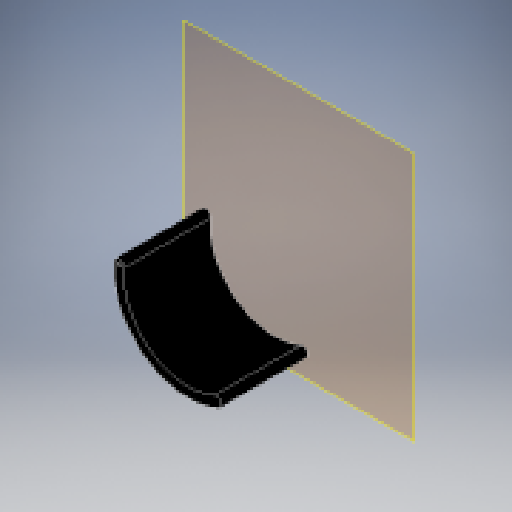
# Autodesk Inventor part: Mesh
Saved by Autodesk Inventor 2026.1 (Build 301233000, 233)
## iProperties
Created: 2025-09-20
Part Number: Mesh
Material: Generic
Document SubType Name: Modeling
Designer: Teddy
Density: 1 g/cm^3
Appearance: Stainless - Satin Coarse Screen
Author: Teddy
Autodesk Inventor part; units mm, degrees
ref_plane "YZ Plane" through (0, 0, 0) normal (1, 0, 0) x (0, 1, 0)
ref_plane "XZ Plane" through (0, 0, 0) normal (0, 1, 0) x (-1, 0, 0)
ref_plane "XY Plane" through (0, 0, 0) normal (0, 0, 1) x (1, 0, 0)
ref_plane "Work Plane1" through (0, 0, 0) normal (0, 0, 1) x (1, 0, 0)
sketch "Sketch1" plane through (0, 0, 0) normal (0, 0, 1) x (1, 0, 0)
  circle A0 centre (-119.9422, -41.6723) radius 2.794 projected
  circle A1 centre (5.1026, -131.5245) radius 2.286 construction
  circle A2 centre (-67.2141, -131.9038) radius 3.9624 construction
  circle A3 centre (-31.4817, -50.501) radius 2.286 projected
  arc A4 (-119.9422, -41.6723) -> (5.1026, -131.5245) centre (-31.4817, -50.501) ccw construction
  arc A5 (-126.2608, -41.0417) -> (7.7158, -137.3119) centre (-31.4817, -50.501) ccw
  arc A6 (-113.6236, -42.3029) -> (2.4895, -125.7371) centre (-31.4817, -50.501) ccw
  arc A7 (-113.6236, -42.3029) -> (-126.2608, -41.0417) centre (-119.9422, -41.6723) ccw
  arc A8 (7.7158, -137.3119) -> (2.4895, -125.7371) centre (5.1026, -131.5245) ccw
  point P0 (0, 0)
  dimension "d0" = 12.7
  constraints: 10 point on circle, 5 centre point, 4 tangent, 1 coincident
  measures "d0" diameter of A8
ref_plane "Work Plane2" through (-268.3983, -269.3131, 111.1682) normal (0, 0, -1) x (0, 1, 0)
extrude "Extrusion1" add sketch "Sketch1" along normal up to surface (111.1682 mm away) contours A7 A6 A8 A5
body "Solid1"
